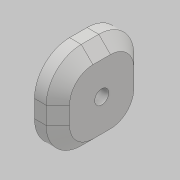
# Autodesk Inventor part: exercise3-1-6
Saved by Autodesk Inventor 2018 (Build 220112000, 112)
## iProperties
Created: 2020-09-21
Part Number: exercise3-1-6
Material: 一般
Document SubType Name: Modeling
Designer: 王鼎鈞
Density: 1 g/cm^3
Appearance: 預設
Author: 王鼎鈞
Autodesk Inventor part; units mm, degrees
ref_plane "YZ Plane" through (0, 0, 0) normal (1, 0, 0) x (0, 1, 0)
ref_plane "XZ Plane" through (0, 0, 0) normal (0, 1, 0) x (-1, 0, 0)
ref_plane "XY Plane" through (0, 0, 0) normal (0, 0, 1) x (1, 0, 0)
sketch "草圖1" plane through (0, 0, 0) normal (1, 0, 0) x (0, 1, 0)
  line L0 (-37.5, 37.5) -> (37.5, 37.5)
  line L1 (37.5, 37.5) -> (37.5, -37.5)
  line L2 (37.5, -37.5) -> (-37.5, -37.5)
  line L3 (-37.5, -37.5) -> (-37.5, 37.5)
  line L4 (-37.5, 37.5) -> (37.5, -37.5) construction
  line L5 (37.5, 37.5) -> (-37.5, -37.5) construction
  point P0 (0, 0)
  dimension "d0" = 75
  dimension "d1" = 75
  constraints: 12 end point, 2 midpoint, 2 parallel, 1 horizontal, 1 perpendicular
  measures "d0" distance of L1.end L2.end
  measures "d1" distance of L0.end L1.end
extrude "擠出1" add sketch "草圖1" along normal blind 20
fillet "圓角1" radius 30 4 edges at (10, 37.5, 37.5) (10, -37.5, 37.5) (10, 37.5, -37.5) (10, -37.5, -37.5)
chamfer "倒角1" distance 10 angle 45 8 edges at (20, 0, 37.5) (20, -28.7132, 28.7132) (20, -37.5, 0) (20, -28.7132, -28.7132) (20, 0, -37.5) (20, 28.7132, -28.7132) (20, 37.5, 0) (20, 28.7132, 28.7132)
sketch "草圖2" plane through (20, 0, 0) normal (1, 0, 0) x (0, 0, -1)
  line L0 (0, 0) -> (0, 0)
  line L1 (0, 0) -> (0, 0)
  line L2 (0, 0) -> (0, 0)
  line L3 (0, 0) -> (0, 0)
  line L4 (0, 0) -> (0, 0) construction
  line L5 (0, 0) -> (0, 0) construction
  point P0 (0, 0)
  dimension "d8" = 0
  dimension "d9" = 0
  constraints: 12 end point, 4 coincident, 2 collinear, 2 midpoint, 1 horizontal, 1 perpendicular
  measures "d8" distance of L2.end L1.end
  measures "d9" distance of L1.end L0.end
hole "孔1" at (20, 0, 0) at (20, 0, 0) at (20, 0, 0) at (20, 0, 0) direction (-1, 0, 0) diameter 12 depth 10 tip angle 118
sketch "草圖3" plane through (0, 0, 0) normal (-1, 0, 0) x (0, 0, 1)
  arc A0 (-37.5, -7.5) -> (-7.5, -37.5) centre (-7.5, -7.5) ccw projected
  line L0 (-7.5, -37.5) -> (7.5, -37.5) projected
  arc A1 (7.5, -37.5) -> (37.5, -7.5) centre (7.5, -7.5) ccw projected
  line L1 (37.5, -7.5) -> (37.5, 7.5) projected
  arc A2 (37.5, 7.5) -> (7.5, 37.5) centre (7.5, 7.5) ccw projected
  line L2 (7.5, 37.5) -> (-7.5, 37.5) projected
  arc A3 (-7.5, 37.5) -> (-37.5, 7.5) centre (-7.5, 7.5) ccw projected
  line L3 (-37.5, 7.5) -> (-37.5, -7.5) projected
  line L4 (12.5, 12.5) -> (-12.5, 12.5)
  line L5 (-12.5, 12.5) -> (-12.5, -12.5)
  line L6 (-12.5, -12.5) -> (12.5, -12.5)
  line L7 (12.5, -12.5) -> (12.5, 12.5)
  line L8 (12.5, 12.5) -> (-12.5, -12.5) construction
  line L9 (-12.5, 12.5) -> (12.5, -12.5) construction
  point P0 (0, 0)
  dimension "d17" = 25
  dimension "d18" = 25
  constraints: 12 end point, 4 coincident, 2 midpoint, 2 parallel, 1 horizontal, 1 perpendicular
  measures "d17" distance of L6.end L5.end
  measures "d18" distance of L5.end L4.end
hole "孔2" at (0, -12.5, 12.5) at (0, -12.5, -12.5) at (0, 12.5, -12.5) at (0, 12.5, 12.5) direction (1, 0, 0) diameter 12 depth 10 tip angle 118
